Autodesk Inventor part; units mm, degrees
(part 2 of 2)
  spline S299 degree 2 poles (22.3623, 53.7806) (22.2981, 54.0029) (22.2339, 54.3685) (22.2339, 54.6451) knots 0 0 0 1 2 2 2
  spline S300 degree 2 poles (25.1337, 53.751) (25.4449, 53.7609) (25.8994, 53.8893) (26.0525, 54.0128) knots 0 0 0 1 2 2 2
  spline S301 degree 2 poles (26.0525, 54.0128) (26.2255, 54.1462) (26.4082, 54.5661) (26.4082, 54.8773) knots 0 0 0 1 2 2 2
  spline S302 degree 2 poles (26.4082, 54.8773) (26.4082, 55.1836) (26.2255, 55.6134) (26.0476, 55.7912) knots 0 0 0 1 2 2 2
  spline S303 degree 2 poles (26.0476, 55.7912) (25.8648, 55.9641) (25.4252, 56.1419) (25.1337, 56.1666) knots 0 0 0 1 2 2 2
  line L176 (25.1337, 56.1666) -> (25.1337, 53.751)
  spline S304 degree 2 poles (24.7484, 48.3861) (23.6023, 48.3861) (22.2487, 49.4778) (22.2487, 50.3127) knots 0 0 0 1 2 2 2
  spline S305 degree 2 poles (22.2487, 50.3127) (22.2487, 50.6536) (22.4068, 51.1772) (22.5698, 51.4489) knots 0 0 0 1 2 2 2
  line L177 (22.5698, 51.4489) -> (20.6531, 51.4489)
  line L178 (20.6531, 51.4489) -> (20.6531, 52.2196)
  line L179 (20.6531, 52.2196) -> (26.9121, 52.2196)
  line L180 (26.9121, 52.2196) -> (26.9121, 51.4489)
  line L181 (26.9121, 51.4489) -> (26.4329, 51.4489)
  spline S306 degree 2 poles (26.4329, 51.4489) (26.6948, 51.1624) (27.0406, 50.4609) (27.0406, 50.0509) knots 0 0 0 1 2 2 2
  spline S307 degree 2 poles (27.0406, 50.0509) (27.0406, 49.2654) (25.7957, 48.3861) (24.7484, 48.3861) knots 0 0 0 1 2 2 2
  spline S308 degree 2 poles (24.6595, 49.1814) (25.4449, 49.1814) (26.3094, 49.6804) (26.3094, 50.2386) knots 0 0 0 1 2 2 2
  spline S309 degree 2 poles (26.3094, 50.2386) (26.3094, 50.5647) (26.018, 51.1772) (25.7907, 51.4489) knots 0 0 0 1 2 2 2
  line L182 (25.7907, 51.4489) -> (23.1923, 51.4489)
  spline S310 degree 2 poles (23.1923, 51.4489) (23.049, 51.1476) (22.9403, 50.7178) (22.9403, 50.4411) knots 0 0 0 1 2 2 2
  spline S311 degree 2 poles (22.9403, 50.4411) (22.9403, 49.8434) (23.8197, 49.1814) (24.6595, 49.1814) knots 0 0 0 1 2 2 2
  spline S312 degree 2 poles (22.2487, 46.2026) (22.2487, 46.83) (22.965, 47.5364) (23.7406, 47.5364) knots 0 0 0 1 2 2 2
  line L183 (23.7406, 47.5364) -> (26.2749, 47.5364)
  line L184 (26.2749, 47.5364) -> (26.2749, 48.0551)
  line L185 (26.2749, 48.0551) -> (26.9121, 48.0551)
  line L186 (26.9121, 48.0551) -> (26.9121, 47.5364)
  line L187 (26.9121, 47.5364) -> (28.2262, 47.5364)
  line L188 (28.2262, 47.5364) -> (28.2262, 46.7658)
  line L189 (28.2262, 46.7658) -> (26.9121, 46.7658)
  line L190 (26.9121, 46.7658) -> (26.9121, 45.348)
  line L191 (26.9121, 45.348) -> (26.2749, 45.348)
  line L192 (26.2749, 45.348) -> (26.2749, 46.7658)
  line L193 (26.2749, 46.7658) -> (24.0963, 46.7658)
  spline S313 degree 2 poles (24.0963, 46.7658) (23.7505, 46.7658) (23.3701, 46.7411) (23.2071, 46.6571) knots 0 0 0 1 2 2 2
  spline S314 degree 2 poles (23.2071, 46.6571) (23.0638, 46.5879) (22.9206, 46.2767) (22.9206, 46.0099) knots 0 0 0 1 2 2 2
  spline S315 degree 2 poles (22.9206, 46.0099) (22.9206, 45.8222) (23.0342, 45.4715) (23.0688, 45.3924) knots 0 0 0 1 2 2 2
  line L194 (23.0688, 45.3924) -> (23.0688, 45.348)
  line L195 (23.0688, 45.348) -> (22.3772, 45.348)
  spline S316 degree 2 poles (22.3772, 45.348) (22.3179, 45.5653) (22.2487, 46.0099) (22.2487, 46.2026) knots 0 0 0 1 2 2 2
  line L196 (22.3376, 38.5159) -> (22.3376, 42.2753)
  line L197 (22.3376, 42.2753) -> (23.2022, 42.2753)
  spline S317 degree 2 poles (23.2022, 42.2753) (23.5825, 41.8702) (24.289, 41.1489) (24.6693, 40.8031) knots 0 0 0 1 2 2 2
  spline S318 degree 2 poles (24.6693, 40.8031) (25.435, 40.1066) (26.3539, 39.5978) (26.843, 39.5978) knots 0 0 0 1 2 2 2
  spline S319 degree 2 poles (26.843, 39.5978) (27.0998, 39.5978) (27.4852, 39.7559) (27.6087, 39.8991) knots 0 0 0 1 2 2 2
  spline S320 degree 2 poles (27.6087, 39.8991) (27.7322, 40.0424) (27.8557, 40.4178) (27.8557, 40.6451) knots 0 0 0 1 2 2 2
  spline S321 degree 2 poles (27.8557, 40.6451) (27.8557, 40.8624) (27.747, 41.307) (27.663, 41.5096) knots 0 0 0 1 2 2 2
  spline S322 degree 2 poles (27.663, 41.5096) (27.5938, 41.6825) (27.3962, 42.0036) (27.3271, 42.1024) knots 0 0 0 1 2 2 2
  line L198 (27.3271, 42.1024) -> (27.3271, 42.1468)
  line L199 (27.3271, 42.1468) -> (28.1965, 42.1468)
  spline S323 degree 2 poles (28.1965, 42.1468) (28.32, 41.8949) (28.5621, 40.9909) (28.5621, 40.5858) knots 0 0 0 1 2 2 2
  spline S324 degree 2 poles (28.5621, 40.5858) (28.5621, 39.7312) (27.6581, 38.7679) (26.8874, 38.7679) knots 0 0 0 1 2 2 2
  spline S325 degree 2 poles (26.8874, 38.7679) (26.5268, 38.7679) (25.9241, 38.9358) (25.6672, 39.084) knots 0 0 0 1 2 2 2
  spline S326 degree 2 poles (25.6672, 39.084) (25.4005, 39.2322) (24.8768, 39.662) (24.6249, 39.8991) knots 0 0 0 1 2 2 2
  spline S327 degree 2 poles (24.6249, 39.8991) (24.205, 40.2844) (23.3059, 41.228) (23.0441, 41.5096) knots 0 0 0 1 2 2 2
  line L200 (23.0441, 41.5096) -> (23.0441, 38.5159)
  line L201 (23.0441, 38.5159) -> (22.3376, 38.5159)
  spline S328 degree 2 poles (25.3856, 33.9069) (23.7456, 33.9069) (22.2092, 34.8603) (22.2092, 35.8532) knots 0 0 0 1 2 2 2
  spline S329 degree 2 poles (22.2092, 35.8532) (22.2092, 36.861) (23.7752, 37.8045) (25.3807, 37.8045) knots 0 0 0 1 2 2 2
  spline S330 degree 2 poles (25.3807, 37.8045) (27.0307, 37.8045) (28.5571, 36.8511) (28.5571, 35.8532) knots 0 0 0 1 2 2 2
  spline S331 degree 2 poles (28.5571, 35.8532) (28.5571, 34.8504) (26.9763, 33.9069) (25.3856, 33.9069) knots 0 0 0 1 2 2 2
  spline S332 degree 2 poles (23.5282, 34.9541) (23.8295, 34.8356) (24.7583, 34.7368) (25.3856, 34.7368) knots 0 0 0 1 2 2 2
  spline S333 degree 2 poles (25.3856, 34.7368) (26.013, 34.7368) (26.9368, 34.8356) (27.248, 34.9591) knots 0 0 0 1 2 2 2
  spline S334 degree 2 poles (27.248, 34.9591) (27.5593, 35.0826) (27.8804, 35.5124) (27.8804, 35.8532) knots 0 0 0 1 2 2 2
  spline S335 degree 2 poles (27.8804, 35.8532) (27.8804, 36.1941) (27.5593, 36.6338) (27.2382, 36.7622) knots 0 0 0 1 2 2 2
  spline S336 degree 2 poles (27.2382, 36.7622) (26.9269, 36.8857) (25.9784, 36.9746) (25.3807, 36.9746) knots 0 0 0 1 2 2 2
  spline S337 degree 2 poles (25.3807, 36.9746) (24.7385, 36.9746) (23.8789, 36.8956) (23.543, 36.7671) knots 0 0 0 1 2 2 2
  spline S338 degree 2 poles (23.543, 36.7671) (23.2269, 36.6486) (22.886, 36.2089) (22.886, 35.8532) knots 0 0 0 1 2 2 2
  spline S339 degree 2 poles (22.886, 35.8532) (22.886, 35.5173) (23.2071, 35.0776) (23.5282, 34.9541) knots 0 0 0 1 2 2 2
  line L202 (22.3376, 29.367) -> (22.3376, 33.1263)
  line L203 (22.3376, 33.1263) -> (23.2022, 33.1263)
  spline S340 degree 2 poles (23.2022, 33.1263) (23.5825, 32.7213) (24.289, 32) (24.6693, 31.6542) knots 0 0 0 1 2 2 2
  spline S341 degree 2 poles (24.6693, 31.6542) (25.435, 30.9577) (26.3539, 30.4488) (26.843, 30.4488) knots 0 0 0 1 2 2 2
  spline S342 degree 2 poles (26.843, 30.4488) (27.0998, 30.4488) (27.4852, 30.6069) (27.6087, 30.7502) knots 0 0 0 1 2 2 2
  spline S343 degree 2 poles (27.6087, 30.7502) (27.7322, 30.8934) (27.8557, 31.2689) (27.8557, 31.4961) knots 0 0 0 1 2 2 2
  spline S344 degree 2 poles (27.8557, 31.4961) (27.8557, 31.7135) (27.747, 32.1581) (27.663, 32.3606) knots 0 0 0 1 2 2 2
  spline S345 degree 2 poles (27.663, 32.3606) (27.5938, 32.5335) (27.3962, 32.8546) (27.3271, 32.9534) knots 0 0 0 1 2 2 2
  line L204 (27.3271, 32.9534) -> (27.3271, 32.9979)
  line L205 (27.3271, 32.9979) -> (28.1965, 32.9979)
  spline S346 degree 2 poles (28.1965, 32.9979) (28.32, 32.746) (28.5621, 31.8419) (28.5621, 31.4368) knots 0 0 0 1 2 2 2
  spline S347 degree 2 poles (28.5621, 31.4368) (28.5621, 30.5822) (27.6581, 29.6189) (26.8874, 29.6189) knots 0 0 0 1 2 2 2
  spline S348 degree 2 poles (26.8874, 29.6189) (26.5268, 29.6189) (25.9241, 29.7869) (25.6672, 29.9351) knots 0 0 0 1 2 2 2
  spline S349 degree 2 poles (25.6672, 29.9351) (25.4005, 30.0833) (24.8768, 30.5131) (24.6249, 30.7502) knots 0 0 0 1 2 2 2
  spline S350 degree 2 poles (24.6249, 30.7502) (24.205, 31.1355) (23.3059, 32.079) (23.0441, 32.3606) knots 0 0 0 1 2 2 2
  line L206 (23.0441, 32.3606) -> (23.0441, 29.367)
  line L207 (23.0441, 29.367) -> (22.3376, 29.367)
  spline S351 degree 2 poles (24.2741, 24.8567) (23.8345, 24.8567) (23.0836, 25.1383) (22.8069, 25.3952) knots 0 0 0 1 2 2 2
  spline S352 degree 2 poles (22.8069, 25.3952) (22.5303, 25.6521) (22.2092, 26.4178) (22.2092, 26.892) knots 0 0 0 1 2 2 2
  spline S353 degree 2 poles (22.2092, 26.892) (22.2092, 27.3267) (22.4019, 28.1764) (22.555, 28.4876) knots 0 0 0 1 2 2 2
  line L208 (22.555, 28.4876) -> (23.4195, 28.4876)
  line L209 (23.4195, 28.4876) -> (23.4195, 28.4284)
  spline S354 degree 2 poles (23.4195, 28.4284) (23.3504, 28.3345) (23.1725, 27.9838) (23.0935, 27.7713) knots 0 0 0 1 2 2 2
  spline S355 degree 2 poles (23.0935, 27.7713) (23.0095, 27.5293) (22.9156, 27.1291) (22.9156, 26.8772) knots 0 0 0 1 2 2 2
  spline S356 degree 2 poles (22.9156, 26.8772) (22.9156, 26.6302) (23.0935, 26.1658) (23.2861, 25.9979) knots 0 0 0 1 2 2 2
  spline S357 degree 2 poles (23.2861, 25.9979) (23.4689, 25.8447) (23.953, 25.6866) (24.2791, 25.6866) knots 0 0 0 1 2 2 2
  spline S358 degree 2 poles (24.2791, 25.6866) (24.6051, 25.6866) (25.0201, 25.8645) (25.1584, 26.0324) knots 0 0 0 1 2 2 2
  spline S359 degree 2 poles (25.1584, 26.0324) (25.3115, 26.2054) (25.44, 26.7191) (25.44, 27.0303) knots 0 0 0 1 2 2 2
  spline S360 degree 2 poles (25.44, 27.0303) (25.44, 27.3663) (25.3362, 28.0332) (25.2918, 28.2357) knots 0 0 0 1 2 2 2
  line L210 (25.2918, 28.2357) -> (28.4336, 28.2357)
  line L211 (28.4336, 28.2357) -> (28.4336, 24.8913)
  line L212 (28.4336, 24.8913) -> (27.7173, 24.8913)
  line L213 (27.7173, 24.8913) -> (27.7173, 27.4502)
  line L214 (27.7173, 27.4502) -> (26.0921, 27.4502)
  spline S361 degree 2 poles (26.0921, 27.4502) (26.1118, 27.302) (26.1267, 27.0155) (26.1267, 26.897) knots 0 0 0 1 2 2 2
  spline S362 degree 2 poles (26.1267, 26.897) (26.1267, 26.4277) (25.9735, 25.7805) (25.7463, 25.4841) knots 0 0 0 1 2 2 2
  spline S363 degree 2 poles (25.7463, 25.4841) (25.519, 25.1828) (24.8274, 24.8567) (24.2741, 24.8567) knots 0 0 0 1 2 2 2
  point P0 (0, 50)
  dimension "d0" = 100
  dimension "d1" = 105
  constraints: 2 other
emboss "Emboss1" sketch "Sketch11" operation cut depth 1.5 direction (0, -1, 0)
mirror "Mirror1" about plane through (0, 0, 0) normal (0, 1, 0) of "Revolution1"
body "Solid1"
